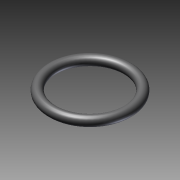
# Autodesk Inventor part: LOCNL2_3
Saved by Autodesk Inventor 2011 SP1 (Build 150282100, 282)
## iProperties
Created: 2015-03-21
Part Number: LOCNL2_3
Catalog Web Link: www.cadenas.de
Description: LOCNL_3-Knuckle Locks
Vendor: MISUMI
Document SubType Name: Modeling
Designer: PARTuser1
Manufacturer: MISUMI
Mass: 0.0197392 g
Surface Area: 0.789568 cm^2
Volume: 0.0197392 cm^3
Density: 1 g/cm^3
Category: PARTsolutions
Company: MISUMI
Title: LOCNL2_3
Author: Cadenas PARTsolutions
Comments: Knuckle Locks
PSOL_IDENT_0: {\\10.0.0.236\data_v8\23d-libs\misumi\metric\44_handles_hinges\locnl_3.prj},159 {VTYP=3D},{NB=LOCNL2
PSOL_IDENT_1: _3},{LINA=LOCNL2_3},{NN=LOCNL_3},{DATE=14.11.2014 09:15:19},{GEOMDATE=09.12.2008 13:44:00},{VERSION=
PSOL_IDENT_2: },{LINEID=20},{LINESUBID=-1},{WBVAR=}  {NB=LOCNL2_3},{LINA=LOCNL2_3},{KT=DUMMY},{PN=LOCNL2},{TYPE=LO
PSOL_IDENT_3: CNL},{MATMB=Zinc Die Casting},{MATHN=Low Carbon Steel},{MATLP=Low Carbon Steel},{MATK=Low Carbon Ste
PSOL_IDENT_4: el},{STMB=Chrome Plating},{STHN=Trivalent Chromate},{STLP=Trivalent Chromate},{STK=Chrome Plating},{
PSOL_IDENT_5: NO=2},{KD=2  Holes},{MASS=25},{AK=2 Pcs.}
SUPPLIER: MISUMI
ARTICLENO: LOCNL2_3
BOMINFO: LOCNL2_3
CREATOR: CADENAS GmbH
Autodesk Inventor part; units mm, degrees
sketch "Sketch_1" plane through (0, 0, 0) normal (1, 0, 0) x (0, 1, 0)
  line L0 (-4, -50) -> (-4, 50)
  circle A0 centre (0, 0) radius 0.5
  constraints: 2 end point, 1 centre point
revolve "Revolution1" add sketch "Sketch_1" angle 360 about axis through (0, -4, -50) along (0, 0, -1)
ref_plane "3_TO_K_XY" through (0, 0, -1) normal (0, 0, 1) x (1, 0, 0)
ref_plane "3_TO_K_YZ" through (0, 0, -1) normal (1, 0, 0) x (0, 1, 0)
ref_plane "3_TO_K_ZX" through (0, 0, -1) normal (0, 1, 0) x (0, 0, 1)
ref_plane "31_TO_K_XY" through (0, -7.5, -1) normal (0, 0, 1) x (1, 0, 0)
ref_plane "31_TO_K_YZ" through (0, -7.5, -1) normal (1, 0, 0) x (0, 1, 0)
ref_plane "31_TO_K_ZX" through (0, -7.5, -1) normal (0, 1, 0) x (0, 0, 1)
body "Solid1"
